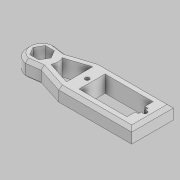
# Autodesk Inventor part: Tibia_V2
Saved by Autodesk Inventor 2022.2 (Build 262287010, 287A)
## iProperties
Created: 2022-06-03
Part Number: Tibia_V2
Material: Genérico
Document SubType Name: Modeling
Designer: Usuario
Density: 1 g/cm^3
Appearance: Valor por defecto
Author: Usuario
Autodesk Inventor part; units mm, degrees
ref_plane "YZ Plane" through (0, 0, 0) normal (1, 0, 0) x (0, 1, 0)
ref_plane "XZ Plane" through (0, 0, 0) normal (0, 1, 0) x (-1, 0, 0)
ref_plane "XY Plane" through (0, 0, 0) normal (0, 0, 1) x (1, 0, 0)
sketch "Boceto1" plane through (0, 0, 0) normal (0, 1, 0) x (-1, 0, 0)
  line L0 (17.5, -10) -> (-17.5, -10)
  line L1 (-17.5, -10) -> (-17.5, 10)
  line L2 (-17.5, 10) -> (17.5, 10)
  line L3 (17.5, 10) -> (17.5, 6.2798) construction
  line L4 (17.5, -10) -> (-17.5, 10) construction
  line L5 (-17.5, -10) -> (17.5, 10) construction
  line L6 (11.5, -6.25) -> (-11.5, -6.25)
  line L7 (-11.5, -6.25) -> (-11.5, 6.25)
  line L8 (-11.5, 6.25) -> (11.5, 6.25)
  line L9 (11.5, 6.25) -> (11.5, -6.25)
  line L10 (11.5, -6.25) -> (-11.5, 6.25) construction
  line L11 (-11.5, -6.25) -> (11.5, 6.25) construction
  arc A0 (36.6767, -6.9004) -> (36.6767, 6.9004) centre (35.5, 0) ccw
  line L12 (42.5, -10) -> (42.5, 4.9137) construction
  line L13 (37.6651, 3.75) -> (39.8301, 0)
  line L14 (39.8301, 0) -> (37.6651, -3.75)
  line L15 (37.6651, -3.75) -> (33.3349, -3.75)
  line L16 (33.3349, -3.75) -> (31.1699, 0)
  line L17 (31.1699, 0) -> (33.3349, 3.75)
  line L18 (33.3349, 3.75) -> (37.6651, 3.75)
  line L19 (28.5244, -2.7519) -> (26.9356, 0)
  line L20 (26.9356, 0) -> (28.5244, 2.7519)
  line L21 (17.5, -6.2798) -> (17.5, -10) construction
  line L22 (17.5, 6.2798) -> (17.5, -6.2798)
  line L23 (36.6767, -6.9004) -> (30, -6)
  line L24 (30, -6) -> (17.5, -10)
  line L25 (36.6767, 6.9004) -> (30, 6)
  line L26 (30, 6) -> (17.5, 10)
  line L27 (17.5, 6.2798) -> (28.5244, 2.7519)
  line L28 (17.5, -6.2798) -> (28.5244, -2.7519)
  point P0 (0, 0)
  point P1 (0, 0)
  point P2 (0, 0)
  point P3 (0, 0)
  point P4 (0, 0)
  point P5 (17.5, 10)
  dimension "d1" = 35
  dimension "d2" = 23
  dimension "d3" = 12.5
  dimension "d4" = 20
  dimension "d6" = 14
  dimension "d7" = 60
  dimension "d8" = 7.5
  dimension "d9" = 0
  dimension "d10" = 3.667
  dimension "d11" = 0
  dimension "d15" = 6
  dimension "d16" = 6
  dimension "d17" = 30
  dimension "d18" = 30
  constraints: 58 end point, 10 parallel, 8 midpoint, 3 horizontal, 2 perpendicular, 2 point on circle, 1 centre point, 1 coincident, 1 tangent, 1 vertical, 13 other
  measures "d1" distance of L0.start L0.end
  measures "d2" distance of L6.start L6.end
  measures "d3" distance of L6.end L7.end
  measures "d4" distance of L0.end L1.end
  measures "d6" diameter of A0
  measures "d7" distance between parallel lines of L12 L1
  measures "d8" distance between parallel lines of L13 L16
  measures "d9" vertical distance of A0.centre point (0, 0)
  measures "d10" distance between parallel lines of L19 L16
  measures "d11" vertical distance of point (0, 0) L19.end
  measures "d15" vertical distance of point (0, 0) L25.end
  measures "d16" vertical distance of point (0, 0) L23.end
  measures "d17" horizontal distance of point (0, 0) L25.end
  measures "d18" horizontal distance of point (0, 0) L23.end
extrude "Extrusión1" add sketch "Boceto1" along normal blind 8
sketch "Boceto2" plane through (0, 8, 0) normal (0, 1, 0) x (1, 0, 0)
  circle A0 centre (-13.85, 0) radius 1
  circle A1 centre (13.85, 0) radius 1
  line L0 (0, 0) -> (0, -2.5102) construction
  dimension "d19" = 2
  dimension "d20" = 2
  dimension "d21" = 27.7
  constraints: 2 centre point, 2 end point, 1 symmetric about line, 1 vertical
  measures "d19" diameter of A0
  measures "d20" diameter of A1
  measures "d21" distance of A1.centre A0.centre
extrude "Extrusión2" cut sketch "Boceto2" against normal through all
sketch "Boceto3" plane through (0, 8, 0) normal (0, 1, 0) x (1, 0, 0)
  line L0 (11.5, 6.25) -> (11.5, -6.25) projected
  line L1 (11.5, 6.25) -> (11.5, -6.25) projected
  line L2 (11.5, 2.3) -> (13, 2.3)
  line L3 (13, 2.3) -> (13, -2.3)
  line L4 (13, -2.3) -> (11.5, -2.3)
  line L5 (11.5, -2.3) -> (11.5, 2.3)
  line L6 (0, 0) -> (1.0594, 0) construction
  point P0 (11.5, 2.3)
  point P1 (11.5, -2.3)
  dimension "d24" = 4.6
  dimension "d34" = 1.5
  constraints: 10 end point, 2 horizontal, 2 parallel, 1 perpendicular, 1 point on line, 1 symmetric about line
  measures "d24" distance between parallel lines of L4 L2
  measures "d34" distance between parallel lines of L0 L3
extrude "Extrusión3" cut sketch "Boceto3" against normal through all
chamfer "Chaflán1" distance 1.5 angle 45 8 edges at (0, 8, -10) (-23.75, 8, -8) (-33.3383, 8, -6.4502) (-42.5, 8, 0) (-33.3383, 8, 6.4502) (-23.75, 8, 8) (0, 8, 10) (17.5, 8, 0)
fillet "Empalme1" radius 6 1 edges at (-26.9356, 4, 0)
chamfer "Chaflán2" distance 1.5 angle 45 8 edges at (0, 0, 10) (17.5, 0, 0) (0, 0, -10) (-23.75, 0, -8) (-33.3383, 0, -6.4502) (-42.5, 0, 0) (-33.3383, 0, 6.4502) (-23.75, 0, 8)
